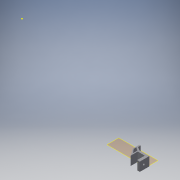
# Autodesk Inventor part: Braces
Saved by Autodesk Inventor 2016 (Build 200138000, 138)
## iProperties
Created: 2016-06-12
Part Number: Braces
Material: Generic
Document SubType Name: Modeling
Designer: Scott
Density: 1 g/cm^3
Appearance: Default
Author: Scott
Autodesk Inventor part; units mm, degrees
ref_plane "YZ Plane" through (0, 0, 0) normal (1, 0, 0) x (0, 1, 0)
ref_plane "XZ Plane" through (0, 0, 0) normal (0, 1, 0) x (-1, 0, 0)
ref_plane "XY Plane" through (0, 0, 0) normal (0, 0, 1) x (1, 0, 0)
ref_plane "Work Plane1" through (330.6234, -207.9752, -19.9742) normal (0, 1, 0) x (-1, 0, -0.0009)
sketch "Sketch1" plane through (330.6234, -207.9752, -19.9742) normal (0, 1, 0) x (-1, 0, -0.0009)
  circle A0 centre (33.1445, -22.86) radius 4 projected
  circle A1 centre (33.1445, -22.86) radius 4 projected
  circle A2 centre (33.1445, -22.86) radius 4 projected
  line L0 (20.4234, -0.007) -> (20.405, 19.993) projected
  line L1 (660.8047, 20.5832) -> (0.405, 19.9746) projected
  line L2 (0.4234, -0.0254) -> (0.405, 19.9746) projected
  line L3 (0.4234, -0.0254) -> (660.8231, 0.5832) projected
  line L4 (660.8047, 20.5832) -> (660.8231, 0.5832) projected
  line L5 (0.405, 19.9746) -> (-7.215, 19.9746)
  line L6 (0.405, 19.9746) -> (0.4234, -0.0254)
  line L7 (0.4234, -0.0254) -> (20.4234, -0.007)
  line L8 (20.4234, -0.007) -> (20.405, 19.993)
  line L9 (35.0462, 0.0065) -> (20.405, 19.993)
  line L10 (-7.215, 19.9746) -> (-7.215, 0.0065)
  line L11 (-7.215, 0.0065) -> (-7.215, -5.0735)
  line L12 (-7.215, -5.0735) -> (20.405, -5.0735)
  line L13 (20.405, -5.0735) -> (31.2395, -11.4268)
  arc A3 (35.0462, -19.341) -> (31.2395, -19.3428) centre (33.1445, -22.86) ccw
  line L14 (31.2395, -19.3428) -> (31.2395, -11.4268)
  line L15 (35.0462, -19.341) -> (35.0462, 0.0065)
  line L16 (20.405, 19.993) -> (20.4234, -0.007)
  line L17 (0.4234, -0.0254) -> (20.4234, -0.007)
  point P0 (330.6048, 20.2789)
  dimension "d0" = 7.62
  dimension "d3" = 5.08
  constraints: 26 end point, 4 collinear, 4 point on circle, 2 perpendicular, 2 point on line, 2 vertical, 1 centre point, 1 horizontal, 1 parallel
  measures "d0" distance of L1.end L5.end
  measures "d3" distance of L10.end L11.end
extrude "Extrusion1" add sketch "Sketch1" along normal blind 25.4 contours A0 L14 L13 L12 L11 L10 L5 L2 L3 L15 | L3 L0 L9
sketch "Sketch2" plane through (337.8431, -207.9752, -25.0411) normal (1, 0, 0.0009) x (0.0009, 0, -1)
  line L0 (14.2693, 0) -> (14.2693, 25.4) projected
  line L1 (-5.0481, 0) -> (-5.0481, 25.4) projected
  line L2 (-25.0481, 25.4) -> (0, 25.4) projected
  line L3 (-25.0481, 0) -> (-25.0481, 25.4) projected
  line L4 (-5.0481, 25.4) -> (-25.0481, 25.4) projected
  line L5 (-15.0481, 25.4) -> (-15.0481, 12.7)
  circle A0 centre (-15.0481, 12.7) radius 2.5
  point P0 (-25.3524, 207.9752)
  dimension "d6" = 5
  constraints: 2 end point, 1 centre point, 1 coincident, 1 midpoint, 1 vertical
  measures "d6" diameter of A0
extrude "Extrusion2" cut sketch "Sketch2" against normal blind 25.4
sketch "Sketch3" plane through (330.6234, -182.5752, -19.9742) normal (0, 1, 0) x (1, 0, 0.0009)
  line L0 (-20.4234, 0.007) -> (-0.4234, 0.0254) projected
  line L1 (-0.4234, 0.0254) -> (-0.405, -19.9746) projected
  line L2 (-0.405, -19.9746) -> (7.215, -19.9746) projected
  line L3 (7.215, -19.9746) -> (7.215, 5.0735) projected
  line L4 (7.215, 5.0735) -> (-20.405, 5.0735) projected
  line L5 (-20.405, 5.0735) -> (-31.2395, 11.4268) projected
  line L6 (-31.2395, 11.4268) -> (-31.2395, 19.3428) projected
  arc A0 (-35.0462, 19.341) -> (-31.2395, 19.3428) centre (-33.1445, 22.86) ccw projected
  line L7 (-35.0462, 19.341) -> (-35.0462, -0.0065) projected
  line L8 (-35.0462, -0.0065) -> (-20.405, -19.993) projected
  line L9 (-20.405, -19.993) -> (-20.4234, 0.007) projected
  line L10 (-32.7964, 8.2501) -> (-32.7964, 0.8179)
  line L11 (-32.7964, 0.8179) -> (-23.4059, -11.0873)
  line L12 (-23.4059, -11.0873) -> (-23.4059, 2.0332)
  line L13 (-23.4059, 2.0332) -> (-32.7964, 8.2501)
  point P0 (-330.6048, -20.2789)
  constraints: 8 end point, 1 parallel, 1 vertical
extrude "Extrusion3" cut sketch "Sketch3" against normal blind 50.8 contours L13 L12 L11 L10
sketch "Sketch4" plane through (337.82, -207.9752, 0.007) normal (-0.0009, 0, 1) x (1, 0, 0.0009)
  point P0 (-337.8199, 207.9752)
sketch "Sketch5" plane through (330.6234, -182.5752, -19.9742) normal (0, 1, 0) x (1, 0, 0.0009)
  line L0 (-0.405, -19.9746) -> (7.215, -19.9746) projected
  line L1 (-0.4234, 0.0254) -> (-0.405, -19.9746) projected
  line L2 (-0.405, -19.9746) -> (-1.675, -19.9746)
  line L3 (-0.405, -19.9746) -> (0.865, -19.9746) construction
  line L4 (-1.675, -19.9746) -> (0.1211, -21.7706)
  line L5 (0.1211, -21.7706) -> (7.215, -21.7706)
  line L6 (7.215, -21.7706) -> (7.215, -19.9746)
  line L7 (-0.405, -19.9746) -> (-0.405, -19.9746)
  line L8 (-0.405, -19.9746) -> (7.215, -19.9746)
  point P0 (-330.6048, -20.2789)
  dimension "d11" = 1.27
  dimension "d12" = 180
  dimension "d13" = 2.54
  dimension "d14" = 45
  constraints: 14 end point, 3 horizontal, 1 collinear, 1 parallel, 1 perpendicular, 1 point on line, 1 vertical
  measures "d11" distance of L0.start L2.end
  measures "d12" angle of L2 L3
  measures "d13" distance of L2.end L4.end
  measures "d14" angle of L4 L2
extrude "Extrusion4" add sketch "Sketch5" against normal up to surface (25.4 mm away)
body "Solid1"
